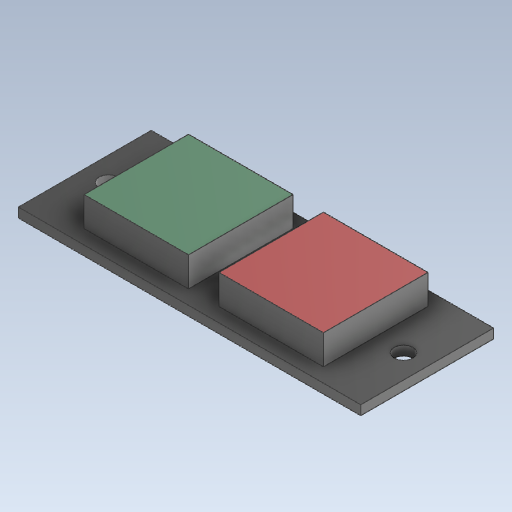
# Autodesk Inventor part: StartStopSwitch
Saved by Autodesk Inventor 2020 (Build 240168000, 168)
## iProperties
Part Number: StartStopSwitch
Material: 一般
Document SubType Name: Modeling
Designer: Masato Kubotera
Density: 1 g/cm^3
Appearance: 滑らか - 黒
Description: CircuitBoard
Author: Masato Kubotera
Autodesk Inventor part; units mm, degrees
ref_plane "YZ Plane" through (0, 0, 0) normal (1, 0, 0) x (0, 1, 0)
ref_plane "XZ Plane" through (0, 0, 0) normal (0, 1, 0) x (-1, 0, 0)
ref_plane "XY Plane" through (0, 0, 0) normal (0, 0, 1) x (1, 0, 0)
derived "Cockpit_top_frame.ipt"
sketch "スケッチ1" plane through (-72.5, 2.5, -22.5) normal (0, 0, 1) x (1, 0, 0)
  line L0 (-7.7, -1.0151) -> (-7.7, 2.5)
  line L1 (-11.725, 2.5) -> (-8.775, 2.5)
  line L2 (-7.7, 2.5) -> (20, 2.5)
  line L3 (20, 2.5) -> (20, -142.5)
  line L4 (20, -70) -> (-12.75, -70) construction
  line L5 (-12.75, -2.5) -> (-12.75, -137.5)
  line L6 (8, 0) -> (0, 0) construction
  line L7 (0, 0) -> (0, -2.5) construction
  line L8 (0, -2.5) -> (8, -2.5) construction
  line L9 (8, -2.5) -> (8, 0) construction
  line L10 (8, 0) -> (0, -2.5) construction
  line L11 (0, 0) -> (8, -2.5) construction
  line L12 (6.5651, 0.05) -> (1.4349, 0.05)
  line L13 (-0.05, -1.4349) -> (-0.05, -2.55)
  line L14 (2.05, -2.55) -> (5.95, -2.55)
  line L15 (8.05, -2.55) -> (8.05, -1.4349)
  line L16 (8.05, 0.05) -> (-0.05, -2.55) construction
  line L17 (-0.05, 0.05) -> (8.05, -2.55) construction
  arc A0 (-0.05, -2.55) -> (2.05, -2.55) centre (1, -2.55) ccw
  arc A1 (1.4349, 0.05) -> (-0.05, -1.4349) centre (0.6925, -0.6925) ccw
  line L18 (4, -2.55) -> (4, 0.05) construction
  arc A2 (5.95, -2.55) -> (8.05, -2.55) centre (7, -2.55) ccw
  arc A3 (8.05, -1.4349) -> (6.5651, 0.05) centre (7.3075, -0.6925) ccw
  circle A4 centre (-4, 0) radius 1.7294 construction
  circle A5 centre (-4, 0) radius 1.6
  circle A6 centre (12, 0) radius 1.7294 construction
  circle A7 centre (12, 0) radius 1.6
  line L19 (-7.75, -2.5) -> (-7.75, 2.5)
  line L20 (0, 2.5) -> (8, 2.5)
  line L21 (-13.5, -2.5) -> (-7.75, -2.5)
  line L22 (-12.75, -137.5) -> (-9.1849, -137.5)
  line L23 (-7.7, -138.9849) -> (-7.7, -142.5)
  line L24 (-7.7, -142.5) -> (20, -142.5)
  circle A8 centre (12, -140) radius 1.6
  circle A9 centre (-4, -140) radius 1.6
  arc A10 (2.05, -137.45) -> (-0.05, -137.45) centre (1, -137.45) ccw
  line L25 (-0.05, -138.5651) -> (-0.05, -137.45)
  arc A11 (-0.05, -138.5651) -> (1.4349, -140.05) centre (0.6925, -139.3075) ccw
  line L26 (6.5651, -140.05) -> (1.4349, -140.05)
  arc A12 (6.5651, -140.05) -> (8.05, -138.5651) centre (7.3075, -139.3075) ccw
  line L27 (8.05, -137.45) -> (8.05, -138.5651)
  arc A13 (8.05, -137.45) -> (5.95, -137.45) centre (7, -137.45) ccw
  line L28 (2.05, -137.45) -> (5.95, -137.45)
  line L29 (-6.75, -41) -> (15.75, -41)
  line L30 (15.75, -41) -> (15.75, -99)
  line L31 (15.75, -99) -> (-6.75, -99)
  line L32 (-6.75, -99) -> (-6.75, -41)
  line L33 (-6.75, -41) -> (15.75, -99) construction
  line L34 (15.75, -41) -> (-6.75, -99) construction
  line L35 (-4.85, -49.22) -> (13.85, -49.22) construction
  line L36 (13.85, -49.22) -> (13.85, -67.92) construction
  line L37 (13.85, -67.92) -> (-4.85, -67.92) construction
  line L38 (-4.85, -67.92) -> (-4.85, -49.22) construction
  line L39 (-4.85, -49.22) -> (13.85, -67.92) construction
  line L40 (13.85, -49.22) -> (-4.85, -67.92) construction
  line L41 (-3.4358, -48.6342) -> (12.4358, -48.6342) construction
  line L42 (14.4358, -50.6342) -> (14.4358, -66.5058) construction
  line L43 (12.4358, -68.5058) -> (-3.4358, -68.5058) construction
  line L44 (-5.4358, -66.5058) -> (-5.4358, -50.6342) construction
  line L45 (-5.4358, -48.6342) -> (14.4358, -68.5058) construction
  line L46 (14.4358, -48.6342) -> (-5.4358, -68.5058) construction
  arc A14 (-5.4358, -66.5058) -> (-3.4358, -68.5058) centre (-3.4358, -66.5058) ccw construction
  arc A15 (12.4358, -68.5058) -> (14.4358, -66.5058) centre (12.4358, -66.5058) ccw construction
  arc A16 (14.4358, -50.6342) -> (12.4358, -48.6342) centre (12.4358, -50.6342) ccw construction
  arc A17 (-3.4358, -48.6342) -> (-5.4358, -50.6342) centre (-3.4358, -50.6342) ccw construction
  line L47 (13.35, -49.72) -> (-4.35, -49.72)
  line L48 (-4.35, -49.72) -> (-4.35, -67.42)
  line L49 (-4.35, -67.42) -> (13.35, -67.42)
  line L50 (13.35, -67.42) -> (13.35, -49.72)
  line L51 (13.35, -49.72) -> (-4.35, -67.42) construction
  line L52 (-4.35, -49.72) -> (13.35, -67.42) construction
  arc A18 (-3.4358, -71.4942) -> (-5.4358, -73.4942) centre (-3.4358, -73.4942) ccw construction
  line L53 (12.4358, -71.4942) -> (-3.4358, -71.4942) construction
  line L54 (-5.4358, -73.4942) -> (-5.4358, -89.3658) construction
  arc A19 (-5.4358, -89.3658) -> (-3.4358, -91.3658) centre (-3.4358, -89.3658) ccw construction
  line L55 (-3.4358, -91.3658) -> (12.4358, -91.3658) construction
  line L56 (14.4358, -89.3658) -> (14.4358, -73.4942) construction
  arc A20 (14.4358, -73.4942) -> (12.4358, -71.4942) centre (12.4358, -73.4942) ccw construction
  line L57 (-5.4358, -91.3658) -> (4.5, -81.43) construction
  line L58 (14.4358, -91.3658) -> (-5.4358, -71.4942) construction
  arc A21 (12.4358, -91.3658) -> (14.4358, -89.3658) centre (12.4358, -89.3658) ccw construction
  line L59 (4.5, -81.43) -> (14.4358, -71.4942) construction
  circle A22 centre (4.5, -45) radius 2 construction
  circle A23 centre (4.5, -45) radius 1.6
  line L60 (-4.35, -90.28) -> (-4.35, -72.58)
  line L61 (-4.35, -72.58) -> (13.35, -72.58)
  line L62 (13.35, -90.28) -> (-4.35, -90.28)
  line L63 (13.35, -72.58) -> (13.35, -90.28)
  circle A24 centre (4.5, -95) radius 2 construction
  circle A25 centre (4.5, -95) radius 1.6
  line L64 (4.5, -99) -> (4.5, -41) construction
  arc A26 (-9.1849, -2.5) -> (-7.7, -1.0151) centre (-8.4425, -1.7575) ccw
  line L65 (-12.75, -2.5) -> (-9.1849, -2.5)
  arc A27 (-7.7, -138.9849) -> (-9.1849, -137.5) centre (-8.4425, -138.2425) ccw
  point P0 (72.5, -2.5)
  point P1 (4, -1.25)
  point P2 (20, -2.5)
  point P3 (4.5, -70)
  point P4 (4.5, -58.57)
  point P5 (4.5, -70)
  point P6 (4.5, -58.57)
  point P7 (15.75, -2.5)
  point P8 (15.75, -2.5)
  point P9 (15.75, -2.5)
  point P10 (-7.7, -2.5)
extrude "押し出し1" add sketch "スケッチ1" against normal blind 1.6 contours L29 L30 L31 L32 | L50 L49 L48 L47 | L60 L61 L63 L62
extrude "押し出し2" add sketch "スケッチ1" along normal blind 5 contours L50 L49 L48 L47 | L60 L61 L63 L62
